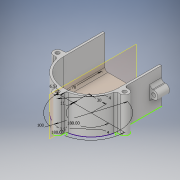
# Autodesk Inventor part: Fej
Saved by Autodesk Inventor 2019 (Build 230136000, 136)
## iProperties
Created: 2020-03-30
Part Number: Fej
Material: Generic
Document SubType Name: Modeling
Designer: laca
Density: 1 g/cm^3
Appearance: Default
Author: laca
Autodesk Inventor part; units mm, degrees
ref_plane "YZ Plane" through (0, 0, 0) normal (1, 0, 0) x (0, 1, 0)
ref_plane "XZ Plane" through (0, 0, 0) normal (0, 1, 0) x (-1, 0, 0)
ref_plane "XY Plane" through (0, 0, 0) normal (0, 0, 1) x (1, 0, 0)
sketch "Sketch1" plane through (0, 0, 0) normal (0, 1, 0) x (-1, 0, 0)
  arc A0 (-10.2866, 48.9304) -> (-48.9304, 10.2866) centre (0, 0) ccw
  circle A1 centre (30, 0) radius 5.5
  circle A2 centre (0, 30) radius 5.5
  circle A3 centre (-30, 0) radius 5.5
  line L0 (50, -11.1096) -> (50, -70)
  line L1 (50, -70) -> (-50, -70)
  line L2 (-50, -70) -> (-50, -11.1096)
  line L3 (-46.5, 0) -> (-46.5, -70)
  line L4 (46.5, -70) -> (46.5, 0)
  arc A4 (46.5, 0) -> (-46.5, 0) centre (0, 0) ccw
  circle A5 centre (57.1096, 0) radius 3.25
  circle A6 centre (57.1096, 0) radius 7.1096
  line L5 (57.1096, -7.1096) -> (54, -7.1096)
  line L6 (57.1096, 7.1096) -> (52.8448, 7.1096)
  circle A7 centre (0, 57.1096) radius 7.1096
  circle A8 centre (0, 57.1096) radius 3.25
  circle A9 centre (-57.1096, 0) radius 7.1096
  circle A10 centre (-57.1096, 0) radius 3.25
  line L7 (-57.1096, -7.1096) -> (-54, -7.1096)
  line L8 (-57.1096, 7.1096) -> (-52.8448, 7.1096)
  line L9 (-7.1096, 57.1096) -> (-7.1096, 52.8448)
  line L10 (7.1096, 57.1096) -> (7.1096, 52.8448)
  arc A11 (48.9304, 10.2866) -> (52.8448, 7.1096) centre (52.8448, 11.1096) ccw
  arc A12 (-52.8448, 7.1096) -> (-48.9304, 10.2866) centre (-52.8448, 11.1096) ccw
  arc A13 (-10.2866, 48.9304) -> (-7.1096, 52.8448) centre (-11.1096, 52.8448) ccw
  arc A14 (54, -7.1096) -> (50, -11.1096) centre (54, -11.1096) ccw
  arc A15 (-50, -11.1096) -> (-54, -7.1096) centre (-54, -11.1096) ccw
  arc A16 (48.9304, 10.2866) -> (10.2866, 48.9304) centre (0, 0) ccw
  arc A17 (7.1096, 52.8448) -> (10.2866, 48.9304) centre (11.1096, 52.8448) ccw
  point P0 (50, 0)
  point P1 (-50, 0)
  point P2 (49.492, 7.1096)
  point P3 (-49.492, 7.1096)
  point P4 (-7.1096, 49.492)
  point P5 (7.1096, 49.492)
  dimension "d0" = 100
  dimension "d1" = 11
  dimension "d2" = 30
  dimension "d5" = 180
  dimension "d7" = 3.5
  dimension "d8" = 70
  dimension "d9" = 6.5
  dimension "d12" = 180
  dimension "d14" = 4
  dimension "d15" = 4
  constraints: 32 point on circle, 22 end point, 18 centre point, 12 tangent, 8 point on line, 5 parallel, 4 equal radius, 4 perpendicular, 2 coincident, 1 vertical, 16 other
  measures "d0" diameter of A0
  measures "d1" diameter of A1
  measures "d2" distance of point (0, 0) A1.centre
  measures "d7" radial gap between concentric circles of A0 A4
  measures "d8" distance from line of L1 point (0, 0)
  measures "d9" diameter of A5
  measures "d14" radius of A11
  measures "d15" radius of A17
extrude "Extrusion1" add sketch "Sketch1" along normal blind 4 contours L3 A4 L4 L1
extrude "Extrusion2" add sketch "Sketch1" along normal blind 60 contours A13 L9 A7 L10 A17 A16 A11 L6 A6 L5 A14 L0 L1 L4 A4 L3 L2 A15 L7 A9 L8 A12 A0 | A7 | A9 | A6
ref_plane "Work Plane1" through (0, 0, -11.1096) normal (1, 0, 0) x (0, 0, -1)
sketch "Sketch2" plane through (50, 0, -70) normal (0, 0, -1) x (-1, 0, 0)
  circle A0 centre (-6.7309, 30) radius 3.25
  arc A1 (-6.7309, 37.25) -> (-6.7309, 22.75) centre (-6.7309, 30) ccw
  line L0 (-6.7309, 37.25) -> (0, 37.25)
  line L1 (0, 0) -> (0, 60) projected
  line L2 (-6.7309, 22.75) -> (0, 22.75)
  line L3 (0, 37.25) -> (0, 22.75)
  line L4 (0, 60) -> (3.5, 60) projected
  point P0 (50, 0)
  dimension "d20" = 6.5
  dimension "d21" = 4
  dimension "d22" = 30
  dimension "d23" = 60
  constraints: 6 end point, 2 centre point, 2 point on circle, 2 point on line, 1 horizontal, 1 parallel, 1 vertical
  measures "d20" diameter of A0
  measures "d21" radial gap between concentric circles of A0 A1
  measures "d22" distance from line of L4 A0.centre
  measures "d23" distance of L1.start L1.end
extrude "Extrusion3" add sketch "Sketch2" against normal blind 20
fillet "Fillet1" radius 5 2 edges at (50, 37.25, -60) (50, 22.75, -60)
mirror "Mirror1" about plane through (0, 0, -11.1096) normal (1, 0, 0) of "Extrusion3"
fillet "Fillet2" radius 5 2 edges at (-50, 37.25, -60) (-50, 22.75, -60)
fillet "Fillet3" radius 5 3 edges at (0, 4, 46.5) (46.5, 4, -35) (-46.5, 4, -35)
equation "\"d22\" = 0.5 * d23"
body "Solid1"
